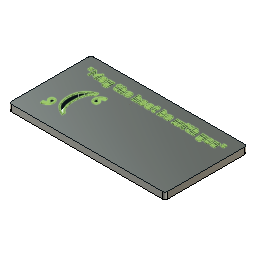
YodaHeatBot_dvirka (Autodesk Fusion 360 design; units mm, degrees)
Autodesk Fusion 360 part; units mm, degrees
(part 1 of 2)
sketch "Sketch1" plane through (0, 0, 0) normal (0, 0, 1) x (1, 0, 0)
  line L0 (-75, 65) -> (39, 65)
  line L1 (41, 63) -> (41, 5)
  line L2 (39, 3) -> (-75, 3)
  line L3 (-77, 5) -> (-77, 63)
  arc A0 (-75, 65) -> (-77, 63) centre (-75, 63) ccw
  arc A1 (41, 63) -> (39, 65) centre (39, 63) ccw
  arc A2 (39, 3) -> (41, 5) centre (39, 5) ccw
  arc A3 (-77, 5) -> (-75, 3) centre (-75, 5) ccw
  point P0 (-77, 65)
  point P1 (41, 65)
  point P2 (-77, 3)
  dimension "d1" = 118
  dimension "d2" = 62
  dimension "d3" = 2
  dimension "d4" = 2
  constraint horizontal L0
  constraint vertical L1
  constraint horizontal L2
  constraint vertical L3
  constraint coincident P0 L0
  constraint coincident P0 L3
  constraint tangent L0 A0
  constraint tangent L3 A0
  constraint coincident P1 L0
  constraint coincident P1 L1
  constraint tangent L0 A1
  constraint tangent L1 A1
  constraint equal A0 A1
  constraint tangent L1 A2
  constraint tangent L2 A2
  constraint equal A0 A2
  constraint coincident P2 L3
  constraint coincident P2 L2
  constraint tangent L3 A3
  constraint tangent L2 A3
  measures "d1" distance of P0 P1
  measures "d2" distance of P0 P2
  measures "d3" radius of A0
  measures "d4" radius of A3
extrude "Extrude1" add sketch "Sketch1" along normal blind 5
sketch "Sketch4" plane through (0, 0, 5) normal (0, 0, 1) x (-1, 0, 0)
  arc A0 (75, -65) -> (77, -63) centre (75, -63) ccw
  line L0 (77, -63) -> (77, -5)
  arc A1 (77, -5) -> (75, -3) centre (75, -5) ccw
  line L1 (75, -3) -> (-39, -3)
  arc A2 (-39, -3) -> (-41, -5) centre (-39, -5) ccw
  line L2 (-41, -5) -> (-41, -63)
  arc A3 (-41, -63) -> (-39, -65) centre (-39, -63) ccw
  line L3 (-39, -65) -> (75, -65)
  line L4 (49.3311, -42.4633) -> (49.3311, -41.8971)
  line L5 (49.3311, -41.8971) -> (49.3311, -41.4334)
  line L6 (49.3311, -41.4334) -> (49.3311, -41.1064)
  line L7 (49.3311, -41.1064) -> (49.3311, -40.8822)
  line L8 (49.3311, -40.8822) -> (49.3311, -40.7324)
  line L9 (49.3311, -40.7324) -> (49.3311, -40.6411)
  line L10 (49.3311, -40.6411) -> (49.3311, -40.6007)
  line L11 (49.3311, -40.6007) -> (49.7704, -40.287)
  line L12 (49.7704, -40.287) -> (50.1824, -39.9549)
  line L13 (50.1824, -39.9549) -> (50.5672, -39.6035)
  line L14 (50.5672, -39.6035) -> (50.9248, -39.2336)
  line L15 (50.9248, -39.2336) -> (51.256, -38.8444)
  line L16 (51.256, -38.8444) -> (51.5592, -38.4367)
  line L17 (51.5592, -38.4367) -> (51.8267, -38.0212)
  line L18 (51.8267, -38.0212) -> (51.8324, -38.0124)
  line L19 (51.8324, -38.0124) -> (52.0854, -37.574)
  line L20 (52.0854, -37.574) -> (52.3183, -37.1206)
  line L21 (52.3183, -37.1206) -> (52.5309, -36.6541)
  line L22 (52.5309, -36.6541) -> (52.7233, -36.1726)
  line L23 (52.7233, -36.1726) -> (52.8964, -35.678)
  line L24 (52.8964, -35.678) -> (53.0369, -35.2137)
  line L25 (53.0369, -35.2137) -> (53.0501, -35.1701)
  line L26 (53.0501, -35.1701) -> (53.1863, -34.6518)
  line L27 (53.1863, -34.6518) -> (53.2378, -34.4225)
  line L28 (53.2378, -34.4225) -> (53.3049, -34.1237)
  line L29 (53.3049, -34.1237) -> (53.4051, -33.5843)
  line L30 (53.4051, -33.5843) -> (53.4885, -33.0343)
  line L31 (53.4885, -33.0343) -> (53.5536, -32.4738)
  line L32 (53.5536, -32.4738) -> (53.6124, -31.9123)
  line L33 (53.6124, -31.9123) -> (53.6599, -31.3465)
  line L34 (53.6599, -31.3465) -> (53.6944, -30.8238)
  line L35 (53.6944, -30.8238) -> (53.6976, -30.7754)
  line L36 (53.6976, -30.7754) -> (53.724, -30.2008)
  line L37 (53.724, -30.2008) -> (53.7398, -29.6201)
  line L38 (53.7398, -29.6201) -> (53.7451, -29.0358)
  line L39 (53.7451, -29.0358) -> (53.7398, -28.4507)
  line L40 (53.7398, -28.4507) -> (53.724, -27.8708)
  line L41 (53.724, -27.8708) -> (53.6976, -27.2953)
  line L42 (53.6976, -27.2953) -> (53.693, -27.2251)
  line L43 (53.693, -27.2251) -> (53.6599, -26.7251)
  line L44 (53.6599, -26.7251) -> (53.6124, -26.1593)
  line L45 (53.6124, -26.1593) -> (53.5536, -25.5979)
  line L46 (53.5536, -25.5979) -> (53.4885, -25.0444)
  line L47 (53.4885, -25.0444) -> (53.4051, -24.5014)
  line L48 (53.4051, -24.5014) -> (53.3049, -23.969)
  line L49 (53.3049, -23.969) -> (53.2269, -23.6264)
  line L50 (53.2269, -23.6264) -> (53.1863, -23.448)
  line L51 (53.1863, -23.448) -> (53.0501, -22.9367)
  line L52 (53.0501, -22.9367) -> (53.0369, -22.8937)
  line L53 (53.0369, -22.8937) -> (52.8964, -22.4359)
  line L54 (52.8964, -22.4359) -> (52.7233, -21.9412)
  line L55 (52.7233, -21.9412) -> (52.5309, -21.4598)
  line L56 (52.5309, -21.4598) -> (52.3183, -20.9932)
  line L57 (52.3183, -20.9932) -> (52.0854, -20.5407)
  line L58 (52.0854, -20.5407) -> (51.8324, -20.1015)
  line L59 (51.8324, -20.1015) -> (51.7849, -20.0277)
  line L60 (51.7849, -20.0277) -> (51.5592, -19.6771)
  line L61 (51.5592, -19.6771) -> (51.256, -19.2633)
  line L62 (51.256, -19.2633) -> (50.9248, -18.8714)
  line L63 (50.9248, -18.8714) -> (50.5672, -18.4998)
  line L64 (50.5672, -18.4998) -> (50.1824, -18.1492)
  line L65 (50.1824, -18.1492) -> (49.7704, -17.8206)
  line L66 (49.7704, -17.8206) -> (49.3311, -17.5131)
  line L67 (49.3311, -17.5131) -> (49.3311, -16.4289)
  line L68 (49.3311, -16.4289) -> (49.3311, -15.6452)
  line L69 (49.3311, -15.6452) -> (50.1253, -15.9809)
  line L70 (50.1253, -15.9809) -> (50.88, -16.3367)
  line L71 (50.88, -16.3367) -> (51.0561, -16.4289)
  line L72 (51.0561, -16.4289) -> (51.5961, -16.7119)
  line L73 (51.5961, -16.7119) -> (52.2735, -17.1072)
  line L74 (52.2735, -17.1072) -> (52.9122, -17.5228)
  line L75 (52.9122, -17.5228) -> (53.0369, -17.6135)
  line L76 (53.0369, -17.6135) -> (53.5114, -17.9586)
  line L77 (53.5114, -17.9586) -> (54.0737, -18.4075)
  line L78 (54.0737, -18.4075) -> (54.6008, -18.8758)
  line L79 (54.6008, -18.8758) -> (55.0928, -19.3643)
  line L80 (55.0928, -19.3643) -> (55.5488, -19.873)
  line L81 (55.5488, -19.873) -> (55.9697, -20.4019)
  line L82 (55.9697, -20.4019) -> (56.3554, -20.951)
  line L83 (56.3554, -20.951) -> (56.7068, -21.5133)
  line L84 (56.7068, -21.5133) -> (57.0249, -22.0967)
  line L85 (57.0249, -22.0967) -> (57.3104, -22.7012)
  line L86 (57.3104, -22.7012) -> (57.5626, -23.3276)
  line L87 (57.5626, -23.3276) -> (57.6636, -23.6264)
  line L88 (57.6636, -23.6264) -> (57.7813, -23.9743)
  line L89 (57.7813, -23.9743) -> (57.9676, -24.6429)
  line L90 (57.9676, -24.6429) -> (58.1231, -25.3247)
  line L91 (58.1231, -25.3247) -> (58.2505, -26.0275)
  line L92 (58.2505, -26.0275) -> (58.3498, -26.7489)
  line L93 (58.3498, -26.7489) -> (58.3954, -27.2251)
  line L94 (58.3954, -27.2251) -> (58.4209, -27.4913)
  line L95 (58.4209, -27.4913) -> (58.4631, -28.2539)
  line L96 (58.4631, -28.2539) -> (58.4772, -29.0358)
  line L97 (58.4772, -29.0358) -> (58.4631, -29.8248)
  line L98 (58.4631, -29.8248) -> (58.4209, -30.5918)
  line L99 (58.4209, -30.5918) -> (58.3988, -30.8238)
  line L100 (58.3988, -30.8238) -> (58.3498, -31.3386)
  line L101 (58.3498, -31.3386) -> (58.2505, -32.0634)
  line L102 (58.2505, -32.0634) -> (58.1231, -32.7672)
  line L103 (58.1231, -32.7672) -> (57.9676, -33.4499)
  line L104 (57.9676, -33.4499) -> (57.7813, -34.1185)
  line L105 (57.7813, -34.1185) -> (57.6789, -34.4225)
  line L106 (57.6789, -34.4225) -> (57.5626, -34.7677)
  line L107 (57.5626, -34.7677) -> (57.3104, -35.3968)
  line L108 (57.3104, -35.3968) -> (57.0249, -36.0057)
  line L109 (57.0249, -36.0057) -> (56.7068, -36.5943)
  line L110 (56.7068, -36.5943) -> (56.3554, -37.1637)
  line L111 (56.3554, -37.1637) -> (55.9697, -37.7119)
  line L112 (55.9697, -37.7119) -> (55.7236, -38.0212)
  line L113 (55.7236, -38.0212) -> (55.5488, -38.2408)
  line L114 (55.5488, -38.2408) -> (55.0928, -38.7495)
  line L115 (55.0928, -38.7495) -> (54.6008, -39.238)
  line L116 (54.6008, -39.238) -> (54.0737, -39.7072)
  line L117 (54.0737, -39.7072) -> (53.5114, -40.1553)
  line L118 (53.5114, -40.1553) -> (53.0369, -40.501)
  line L119 (53.0369, -40.501) -> (52.9122, -40.5919)
  line L120 (52.9122, -40.5919) -> (52.2735, -41.0092)
  line L121 (52.2735, -41.0092) -> (51.5961, -41.4072)
  line L122 (51.5961, -41.4072) -> (50.88, -41.7868)
  line L123 (50.88, -41.7868) -> (50.1253, -42.1479)
  line L124 (50.1253, -42.1479) -> (49.3311, -42.4897)
  line L125 (49.3311, -42.4897) -> (49.3311, -42.4633)
  line L126 (64.1054, -21.6205) -> (64.0263, -21.8358)
  line L127 (64.0263, -21.8358) -> (63.92, -22.0273)
  line L128 (63.92, -22.0273) -> (63.8331, -22.1381)
  line L129 (63.8331, -22.1381) -> (63.7882, -22.1951)
  line L130 (63.7882, -22.1951) -> (63.6301, -22.3392)
  line L131 (63.6301, -22.3392) -> (63.4474, -22.464)
  line L132 (63.4474, -22.464) -> (63.2523, -22.5633)
  line L133 (63.2523, -22.5633) -> (63.0467, -22.6379)
  line L134 (63.0467, -22.6379) -> (62.8297, -22.688)
  line L135 (62.8297, -22.688) -> (62.6013, -22.7126)
  line L136 (62.6013, -22.7126) -> (62.3614, -22.7126)
  line L137 (62.3614, -22.7126) -> (62.0337, -22.6753)
  line L138 (62.0337, -22.6753) -> (62.0293, -22.6748)
  line L139 (62.0293, -22.6748) -> (61.7218, -22.5984)
  line L140 (61.7218, -22.5984) -> (61.4407, -22.4833)
  line L141 (61.4407, -22.4833) -> (61.185, -22.3296)
  line L142 (61.185, -22.3296) -> (60.9548, -22.1371)
  line L143 (60.9548, -22.1371) -> (60.7492, -21.9061)
  line L144 (60.7492, -21.9061) -> (60.5752, -21.6425)
  line L145 (60.5752, -21.6425) -> (60.4364, -21.3499)
  line L146 (60.4364, -21.3499) -> (60.3336, -21.031)
  line L147 (60.3336, -21.031) -> (60.266, -20.6848)
  line L148 (60.266, -20.6848) -> (60.2344, -20.3106)
  line L149 (60.2344, -20.3106) -> (60.2368, -20.0277)
  line L150 (60.2368, -20.0277) -> (60.2379, -19.909)
  line L151 (60.2379, -19.909) -> (60.259, -19.6534)
  line L152 (60.259, -19.6534) -> (60.2923, -19.4012)
  line L153 (60.2923, -19.4012) -> (60.3398, -19.1535)
  line L154 (60.3398, -19.1535) -> (60.4004, -18.9083)
  line L155 (60.4004, -18.9083) -> (60.4742, -18.6676)
  line L156 (60.4742, -18.6676) -> (60.5621, -18.4304)
  line L157 (60.5621, -18.4304) -> (60.6505, -18.2283)
  line L158 (60.6505, -18.2283) -> (60.664, -18.1976)
  line L159 (60.664, -18.1976) -> (60.78, -17.9726)
  line L160 (60.78, -17.9726) -> (60.91, -17.753)
  line L161 (60.91, -17.753) -> (61.0541, -17.5412)
  line L162 (61.0541, -17.5412) -> (61.2131, -17.3348)
  line L163 (61.2131, -17.3348) -> (61.3862, -17.1362)
  line L164 (61.3862, -17.1362) -> (61.5812, -16.9438)
  line L165 (61.5812, -16.9438) -> (61.7912, -16.7584)
  line L166 (61.7912, -16.7584) -> (62.0188, -16.5801)
  line L167 (62.0188, -16.5801) -> (62.0337, -16.5695)
  line L168 (62.0337, -16.5695) -> (62.2316, -16.4289)
  line L169 (62.2316, -16.4289) -> (62.2613, -16.4079)
  line L170 (62.2613, -16.4079) -> (62.5213, -16.2427)
  line L171 (62.5213, -16.2427) -> (62.7963, -16.0837)
  line L172 (62.7963, -16.0837) -> (63.095, -15.9405)
  line L173 (63.095, -15.9405) -> (63.4113, -15.8069)
  line L174 (63.4113, -15.8069) -> (63.7461, -15.6848)
  line L175 (63.7461, -15.6848) -> (64.0984, -15.5732)
  line L176 (64.0984, -15.5732) -> (64.4683, -15.4722)
  line L177 (64.4683, -15.4722) -> (64.8566, -15.3826)
  line L178 (64.8566, -15.3826) -> (64.802, -16.4289)
  line L179 (64.802, -16.4289) -> (64.7939, -16.5848)
  line L180 (64.7939, -16.5848) -> (64.7932, -16.5985)
  line L181 (64.7932, -16.5985) -> (64.7924, -16.6144)
  line L182 (64.7924, -16.6144) -> (64.7916, -16.6285)
  line L183 (64.7916, -16.6285) -> (64.7912, -16.6367)
  line L184 (64.7912, -16.6367) -> (64.7908, -16.6436)
  line L185 (64.7908, -16.6436) -> (64.7907, -16.646)
  line L186 (64.7907, -16.646) -> (64.615, -16.7013)
  line L187 (64.615, -16.7013) -> (64.4463, -16.7567)
  line L188 (64.4463, -16.7567) -> (64.2846, -16.8129)
  line L189 (64.2846, -16.8129) -> (64.13, -16.8691)
  line L190 (64.13, -16.8691) -> (63.9815, -16.9262)
  line L191 (63.9815, -16.9262) -> (63.8401, -16.9833)
  line L192 (63.8401, -16.9833) -> (63.8331, -16.9863)
  line L193 (63.8331, -16.9863) -> (63.7118, -17.0369)
  line L194 (63.7118, -17.0369) -> (63.5879, -17.0932)
  line L195 (63.5879, -17.0932) -> (63.4711, -17.1529)
  line L196 (63.4711, -17.1529) -> (63.3586, -17.2162)
  line L197 (63.3586, -17.2162) -> (63.2532, -17.2821)
  line L198 (63.2532, -17.2821) -> (63.1854, -17.3286)
  line L199 (63.1854, -17.3286) -> (63.1521, -17.3515)
  line L200 (63.1521, -17.3515) -> (63.0643, -17.4191)
  line L201 (63.0643, -17.4191) -> (62.9826, -17.4912)
  line L202 (62.9826, -17.4912) -> (62.9079, -17.5676)
  line L203 (62.9079, -17.5676) -> (62.8394, -17.6484)
  line L204 (62.8394, -17.6484) -> (62.7779, -17.7328)
  line L205 (62.7779, -17.7328) -> (62.7234, -17.8224)
  line L206 (62.7234, -17.8224) -> (62.6751, -17.9103)
  line L207 (62.6751, -17.9103) -> (62.6355, -18.0034)
  line L208 (62.6355, -18.0034) -> (62.603, -18.1018)
  line L209 (62.603, -18.1018) -> (62.5775, -18.2055)
  line L210 (62.5775, -18.2055) -> (62.574, -18.2283)
  line L211 (62.574, -18.2283) -> (62.5609, -18.3144)
  line L212 (62.5609, -18.3144) -> (62.5503, -18.4286)
  line L213 (62.5503, -18.4286) -> (62.5503, -18.5033)
  line L214 (62.5503, -18.5033) -> (62.5582, -18.5736)
  line L215 (62.5582, -18.5736) -> (62.5749, -18.6412)
  line L216 (62.5749, -18.6412) -> (62.5986, -18.7054)
  line L217 (62.5986, -18.7054) -> (62.6303, -18.7651)
  line L218 (62.6303, -18.7651) -> (62.6707, -18.8222)
  line L219 (62.6707, -18.8222) -> (62.712, -18.8705)
  line L220 (62.712, -18.8705) -> (62.7577, -18.9189)
  line L221 (62.7577, -18.9189) -> (62.8086, -18.9654)
  line L222 (62.8086, -18.9654) -> (62.864, -19.012)
  line L223 (62.864, -19.012) -> (62.8834, -19.0266)
  line L224 (62.8834, -19.0266) -> (62.9246, -19.0577)
  line L225 (62.9246, -19.0577) -> (62.9905, -19.1025)
  line L226 (62.9905, -19.1025) -> (63.0265, -19.128)
  line L227 (63.0265, -19.128) -> (63.0537, -19.1473)
  line L228 (63.0537, -19.1473) -> (63.072, -19.1604)
  line L229 (63.072, -19.1604) -> (63.1188, -19.1939)
  line L230 (63.1188, -19.1939) -> (63.1855, -19.2404)
  line L231 (63.1855, -19.2404) -> (63.2273, -19.2699)
  line L232 (63.2273, -19.2699) -> (63.2541, -19.2888)
  line L233 (63.2541, -19.2888) -> (63.3252, -19.338)
  line L234 (63.3252, -19.338) -> (63.3973, -19.388)
  line L235 (63.3973, -19.388) -> (63.4702, -19.4408)
  line L236 (63.4702, -19.4408) -> (63.5405, -19.497)
  line L237 (63.5405, -19.497) -> (63.609, -19.5576)
  line L238 (63.609, -19.5576) -> (63.6749, -19.6217)
  line L239 (63.6749, -19.6217) -> (63.739, -19.6894)
  line L240 (63.739, -19.6894) -> (63.8005, -19.7614)
  line L241 (63.8005, -19.7614) -> (63.8331, -19.8002)
  line L242 (63.8331, -19.8002) -> (63.8647, -19.8379)
  line L243 (63.8647, -19.8379) -> (63.9227, -19.9205)
  line L244 (63.9227, -19.9205) -> (63.9763, -20.0083)
  line L245 (63.9763, -20.0083) -> (63.9863, -20.0277)
  line L246 (63.9863, -20.0277) -> (64.0246, -20.1015)
  line L247 (64.0246, -20.1015) -> (64.0685, -20.2007)
  line L248 (64.0685, -20.2007) -> (64.1063, -20.3053)
  line L249 (64.1063, -20.3053) -> (64.1379, -20.4169)
  line L250 (64.1379, -20.4169) -> (64.1625, -20.539)
  line L251 (64.1625, -20.539) -> (64.1792, -20.6699)
  line L252 (64.1792, -20.6699) -> (64.1889, -20.8096)
  line L253 (64.1889, -20.8096) -> (64.1915, -20.9598)
  line L254 (64.1915, -20.9598) -> (64.1871, -21.1189)
  line L255 (64.1871, -21.1189) -> (64.159, -21.3816)
  line L256 (64.159, -21.3816) -> (64.1054, -21.6205)
  line L257 (46.9466, -38.7091) -> (46.8851, -38.9533)
  line L258 (46.8851, -38.9533) -> (46.8095, -39.195)
  line L259 (46.8095, -39.195) -> (46.7199, -39.4322)
  line L260 (46.7199, -39.4322) -> (46.6162, -39.6632)
  line L261 (46.6162, -39.6632) -> (46.4976, -39.889)
  line L262 (46.4976, -39.889) -> (46.3641, -40.1087)
  line L263 (46.3641, -40.1087) -> (46.2165, -40.3222)
  line L264 (46.2165, -40.3222) -> (46.0539, -40.5304)
  line L265 (46.0539, -40.5304) -> (45.8703, -40.7325)
  line L266 (45.8703, -40.7325) -> (45.8395, -40.7624)
  line L267 (45.8395, -40.7624) -> (45.6691, -40.9284)
  line L268 (45.6691, -40.9284) -> (45.4521, -41.1191)
  line L269 (45.4521, -41.1191) -> (45.2184, -41.3036)
  line L270 (45.2184, -41.3036) -> (44.968, -41.4819)
  line L271 (44.968, -41.4819) -> (44.7551, -41.6199)
  line L272 (44.7551, -41.6199) -> (44.7009, -41.655)
  line L273 (44.7009, -41.655) -> (44.4101, -41.814)
  line L274 (44.4101, -41.814) -> (44.1017, -41.9634)
  line L275 (44.1017, -41.9634) -> (43.774, -42.1031)
  line L276 (43.774, -42.1031) -> (43.4278, -42.2331)
  line L277 (43.4278, -42.2331) -> (43.0632, -42.3526)
  line L278 (43.0632, -42.3526) -> (42.6801, -42.4633)
  line L279 (42.6801, -42.4633) -> (42.6801, -41.6199)
  line L280 (42.6801, -41.6199) -> (42.6801, -41.4417)
  line L281 (42.6801, -41.4417) -> (42.6801, -41.3678)
  line L282 (42.6801, -41.3678) -> (42.6801, -41.3073)
  line L283 (42.6801, -41.3073) -> (42.6801, -41.2544)
  line L284 (42.6801, -41.2544) -> (42.6801, -41.2446)
  line L285 (42.6801, -41.2446) -> (42.6801, -41.2315)
  line L286 (42.6801, -41.2315) -> (42.6801, -41.2143)
  line L287 (42.6801, -41.2143) -> (42.6801, -41.2051)
  line L288 (42.6801, -41.2051) -> (42.6801, -41.2018)
  line L289 (42.6801, -41.2018) -> (42.6801, -41.1981)
  line L290 (42.6801, -41.1981) -> (42.8523, -41.134)
  line L291 (42.8523, -41.134) -> (43.0175, -41.069)
  line L292 (43.0175, -41.069) -> (43.1765, -41.0049)
  line L293 (43.1765, -41.0049) -> (43.3285, -40.9407)
  line L294 (43.3285, -40.9407) -> (43.4735, -40.8757)
  line L295 (43.4735, -40.8757) -> (43.6114, -40.8116)
  line L296 (43.6114, -40.8116) -> (43.7371, -40.7518)
  line L297 (43.7371, -40.7518) -> (43.8574, -40.6886)
  line L298 (43.8574, -40.6886) -> (43.9717, -40.6227)
  line L299 (43.9717, -40.6227) -> (44.0402, -40.5792)
  line L300 (44.0402, -40.5792) -> (44.0797, -40.5541)
  line L301 (44.0797, -40.5541) -> (44.1825, -40.4821)
  line L302 (44.1825, -40.4821) -> (44.2792, -40.4074)
  line L303 (44.2792, -40.4074) -> (44.3635, -40.3354)
  line L304 (44.3635, -40.3354) -> (44.4408, -40.2589)
  line L305 (44.4408, -40.2589) -> (44.512, -40.179)
  line L306 (44.512, -40.179) -> (44.5761, -40.0946)
  line L307 (44.5761, -40.0946) -> (44.6332, -40.0068)
  line L308 (44.6332, -40.0068) -> (44.6833, -39.9154)
  line L309 (44.6833, -39.9154) -> (44.7264, -39.8249)
  line L310 (44.7264, -39.8249) -> (44.728, -39.8205)
  line L311 (44.728, -39.8205) -> (44.7615, -39.73)
  line L312 (44.7615, -39.73) -> (44.7887, -39.6299)
  line L313 (44.7887, -39.6299) -> (44.8081, -39.5253)
  line L314 (44.8081, -39.5253) -> (44.8204, -39.4155)
  line L315 (44.8204, -39.4155) -> (44.8239, -39.3004)
  line L316 (44.8239, -39.3004) -> (44.8204, -39.2266)
  line L317 (44.8204, -39.2266) -> (44.8081, -39.1563)
  line L318 (44.8081, -39.1563) -> (44.7887, -39.0895)
  line L319 (44.7887, -39.0895) -> (44.7615, -39.0271)
  line L320 (44.7615, -39.0271) -> (44.7264, -38.9683)
  line L321 (44.7264, -38.9683) -> (44.6889, -38.9208)
  line L322 (44.6889, -38.9208) -> (44.6833, -38.9138)
  line L323 (44.6833, -38.9138) -> (44.6403, -38.8672)
  line L324 (44.6403, -38.8672) -> (44.5919, -38.8224)
  line L325 (44.5919, -38.8224) -> (44.5384, -38.7776)
  line L326 (44.5384, -38.7776) -> (44.4804, -38.7346)
  line L327 (44.4804, -38.7346) -> (44.454, -38.7166)
  line L328 (44.454, -38.7166) -> (44.4395, -38.7067)
  line L329 (44.4395, -38.7067) -> (44.4171, -38.6915)
  line L330 (44.4171, -38.6915) -> (44.3579, -38.6554)
  line L331 (44.3579, -38.6554) -> (44.3495, -38.6502)
  line L332 (44.3495, -38.6502) -> (44.3199, -38.6315)
  line L333 (44.3199, -38.6315) -> (44.2844, -38.6089)
  line L334 (44.2844, -38.6089) -> (44.2168, -38.5659)
  line L335 (44.2168, -38.5659) -> (44.1474, -38.5228)
  line L336 (44.1474, -38.5228) -> (44.0762, -38.478)
  line L337 (44.0762, -38.478) -> (44.0402, -38.4559)
  line L338 (44.0402, -38.4559) -> (44.0033, -38.4332)
  line L339 (44.0033, -38.4332) -> (43.9277, -38.3867)
  line L340 (43.9277, -38.3867) -> (43.8522, -38.3375)
  line L341 (43.8522, -38.3375) -> (43.7792, -38.2847)
  line L342 (43.7792, -38.2847) -> (43.7081, -38.2285)
  line L343 (43.7081, -38.2285) -> (43.6387, -38.1679)
  line L344 (43.6387, -38.1679) -> (43.571, -38.1038)
  line L345 (43.571, -38.1038) -> (43.506, -38.0352)
  line L346 (43.506, -38.0352) -> (43.493, -38.0212)
  line L347 (43.493, -38.0212) -> (43.4384, -37.9623)
  line L348 (43.4384, -37.9623) -> (43.3751, -37.8832)
  line L349 (43.3751, -37.8832) -> (43.3171, -37.798)
  line L350 (43.3171, -37.798) -> (43.2635, -37.7075)
  line L351 (43.2635, -37.7075) -> (43.2152, -37.6109)
  line L352 (43.2152, -37.6109) -> (43.1721, -37.5081)
  line L353 (43.1721, -37.5081) -> (43.1344, -37.3974)
  line L354 (43.1344, -37.3974) -> (43.1036, -37.2779)
  line L355 (43.1036, -37.2779) -> (43.0799, -37.1478)
  line L356 (43.0799, -37.1478) -> (43.0632, -37.0082)
  line L357 (43.0632, -37.0082) -> (43.0527, -36.8588)
  line L358 (43.0527, -36.8588) -> (43.0491, -36.6998)
  line L359 (43.0491, -36.6998) -> (43.0632, -36.4353)
  line L360 (43.0632, -36.4353) -> (43.0989, -36.2218)
  line L361 (43.0989, -36.2218) -> (43.1036, -36.1937)
  line L362 (43.1036, -36.1937) -> (43.1721, -35.9749)
  line L363 (43.1721, -35.9749) -> (43.2679, -35.7781)
  line L364 (43.2679, -35.7781) -> (43.3909, -35.6042)
  line L365 (43.3909, -35.6042) -> (43.5412, -35.4522)
  line L366 (43.5412, -35.4522) -> (43.7177, -35.3177)
  line L367 (43.7177, -35.3177) -> (43.9066, -35.2079)
  line L368 (43.9066, -35.2079) -> (44.0402, -35.1514)
  line L369 (44.0402, -35.1514) -> (44.1078, -35.1227)
  line L370 (44.1078, -35.1227) -> (44.3222, -35.0621)
  line L371 (44.3222, -35.0621) -> (44.5489, -35.0252)
  line L372 (44.5489, -35.0252) -> (44.7887, -35.0129)
  line L373 (44.7887, -35.0129) -> (45.1226, -35.0331)
  line L374 (45.1226, -35.0331) -> (45.4328, -35.0928)
  line L375 (45.4328, -35.0928) -> (45.7201, -35.193)
  line L376 (45.7201, -35.193) -> (45.8395, -35.2563)
  line L377 (45.8395, -35.2563) -> (45.9836, -35.3327)
  line L378 (45.9836, -35.3327) -> (46.2235, -35.5128)
  line L379 (46.2235, -35.5128) -> (46.4405, -35.7333)
  line L380 (46.4405, -35.7333) -> (46.6285, -35.9881)
  line L381 (46.6285, -35.9881) -> (46.7823, -36.2719)
  line L382 (46.7823, -36.2719) -> (46.9018, -36.5856)
  line L383 (46.9018, -36.5856) -> (46.987, -36.9282)
  line L384 (46.987, -36.9282) -> (47.0388, -37.2998)
  line L385 (47.0388, -37.2998) -> (47.0555, -37.7014)
  line L386 (47.0555, -37.7014) -> (47.0485, -37.9579)
  line L387 (47.0485, -37.9579) -> (47.0434, -38.0212)
  line L388 (47.0434, -38.0212) -> (47.0283, -38.2109)
  line L389 (47.0283, -38.2109) -> (46.994, -38.4613)
  line L390 (46.994, -38.4613) -> (46.9466, -38.7091)
  line L391 (68.8125, -55.0356) -> (68.8125, -56.7856)
  line L392 (68.8125, -56.7856) -> (68.2315, -56.7856)
  line L393 (68.2315, -56.7856) -> (68.2315, -55.0356)
  line L394 (68.2315, -55.0356) -> (68.8125, -55.0356)
  line L395 (67.6505, -55.0356) -> (67.6505, -56.7856)
  line L396 (67.6505, -56.7856) -> (67.0625, -56.7856)
  line L397 (67.0625, -56.7856) -> (67.0625, -55.0356)
  line L398 (67.0625, -55.0356) -> (67.6505, -55.0356)
  line L399 (65.3195, -51.5356) -> (65.3195, -56.7856)
  line L400 (65.3195, -56.7856) -> (65.0465, -56.7856)
  line L401 (65.0465, -56.7856) -> (62.5545, -54.3006)
  line L402 (62.5545, -54.3006) -> (60.0695, -56.7856)
  line L403 (60.0695, -56.7856) -> (59.4815, -56.7856)
  line L404 (59.4815, -56.7856) -> (59.4815, -51.5356)
  line L405 (59.4815, -51.5356) -> (60.6505, -51.5356)
  line L406 (60.6505, -51.5356) -> (60.6505, -54.7416)
  line L407 (60.6505, -54.7416) -> (62.6945, -52.6976)
  line L408 (62.6945, -52.6976) -> (64.7315, -54.7416)
  line L409 (64.7315, -54.7416) -> (64.7315, -51.5356)
  line L410 (64.7315, -51.5356) -> (65.3195, -51.5356)
  line L411 (55.9815, -53.8666) -> (55.9815, -54.4546)
  spline S0 degree 3 poles (55.9815, -54.4546) (55.9889, -54.5312) (56.0039, -54.6852) (56.1055, -54.8019) (56.1565, -54.8606) knots 0 0 0 0 0.02248 0.045204 0.045204 0.045204 0.045204
  spline S1 degree 3 poles (56.1565, -54.8606) (56.2158, -54.9117) (56.3348, -55.0141) (56.4911, -55.0284) (56.5695, -55.0356) knots 0 0 0 0 0.022867 0.045862 0.045862 0.045862 0.045862
  line L412 (56.5695, -55.0356) -> (57.1505, -55.0356)
  spline S2 degree 3 poles (57.1505, -55.0356) (57.3046, -55.0073) (57.6273, -54.9481) (57.6957, -54.624) (57.7315, -54.4546) knots 0 0 0 0 0.042955 0.089979 0.089979 0.089979 0.089979
  line L413 (57.7315, -54.4546) -> (58.3195, -54.4546)
  spline S3 degree 3 poles (58.3195, -54.4546) (58.2447, -54.7933) (58.1018, -55.4397) (57.4573, -55.5596) (57.1505, -55.6166) knots 0 0 0 0 0.094379 0.180125 0.180125 0.180125 0.180125
  line L414 (57.1505, -55.6166) -> (55.9815, -55.6166)
  spline S4 degree 3 poles (55.9815, -55.6166) (55.8281, -55.6021) (55.5196, -55.5727) (55.2819, -55.3737) (55.1625, -55.2736) knots 0 0 0 0 0.045098 0.090676 0.090676 0.090676 0.090676
  spline S5 degree 3 poles (55.1625, -55.2736) (55.0625, -55.1542) (54.8634, -54.9166) (54.8341, -54.6081) (54.8195, -54.4546) knots 0 0 0 0 0.045579 0.090676 0.090676 0.090676 0.090676
  line L415 (54.8195, -54.4546) -> (54.8195, -51.5356)
  line L416 (54.8195, -51.5356) -> (55.9815, -51.5356)
  line L417 (55.9815, -51.5356) -> (55.9815, -52.1166)
  spline S6 degree 3 poles (55.9815, -52.1166) (56.0193, -51.9473) (56.0916, -51.6233) (56.4151, -51.564) (56.5695, -51.5356) knots 0 0 0 0 0.047223 0.090343 0.090343 0.090343 0.090343
  line L418 (56.5695, -51.5356) -> (57.1505, -51.5356)
  spline S7 degree 3 poles (57.1505, -51.5356) (57.3044, -51.5504) (57.6147, -51.5801) (57.8552, -51.7786) (57.9765, -51.8786) knots 0 0 0 0 0.04527 0.091283 0.091283 0.091283 0.091283
  spline S8 degree 3 poles (57.9765, -51.8786) (58.0765, -51.9987) (58.2764, -52.2386) (58.3051, -52.5494) (58.3195, -52.7046) knots 0 0 0 0 0.045723 0.091337 0.091337 0.091337 0.091337
  spline S9 degree 3 poles (58.3195, -52.7046) (58.3049, -52.8581) (58.2756, -53.1666) (58.0765, -53.4042) (57.9765, -53.5236) knots 0 0 0 0 0.045098 0.090676 0.090676 0.090676 0.090676
  spline S10 degree 3 poles (57.9765, -53.5236) (57.8552, -53.6237) (57.6147, -53.8222) (57.3044, -53.8519) (57.1505, -53.8666) knots 0 0 0 0 0.046013 0.091283 0.091283 0.091283 0.091283
  line L419 (57.1505, -53.8666) -> (55.9815, -53.8666)
  line L420 (55.9815, -53.2856) -> (56.5695, -53.2856)
  spline S11 degree 3 poles (56.5695, -53.2856) (56.6465, -53.278) (56.8023, -53.2627) (56.922, -53.1617) (56.9825, -53.1106) knots 0 0 0 0 0.022652 0.045806 0.045806 0.045806 0.045806
  spline S12 degree 3 poles (56.9825, -53.1106) (57.0315, -53.0517) (57.1295, -52.9338) (57.1435, -52.7811) (57.1505, -52.7046) knots 0 0 0 0 0.022425 0.044871 0.044871 0.044871 0.044871
  spline S13 degree 3 poles (57.1505, -52.7046) (57.1433, -52.6278) (57.129, -52.4732) (57.0315, -52.3524) (56.9825, -52.2916) knots 0 0 0 0 0.022618 0.045479 0.045479 0.045479 0.045479
  spline S14 degree 3 poles (56.9825, -52.2916) (56.922, -52.2406) (56.8023, -52.1396) (56.6465, -52.1243) (56.5695, -52.1166) knots 0 0 0 0 0.023154 0.045806 0.045806 0.045806 0.045806
  spline S15 degree 3 poles (56.5695, -52.1166) (56.4911, -52.1239) (56.3348, -52.1382) (56.2158, -52.2406) (56.1565, -52.2916) knots 0 0 0 0 0.022995 0.045862 0.045862 0.045862 0.045862
  spline S16 degree 3 poles (56.1565, -52.2916) (56.1055, -52.3522) (56.0045, -52.4719) (55.9891, -52.6276) (55.9815, -52.7046) knots 0 0 0 0 0.023154 0.045806 0.045806 0.045806 0.045806
  line L421 (55.9815, -52.7046) -> (55.9815, -53.2856)
  spline S17 degree 3 poles (53.0625, -50.9546) (53.031, -50.7832) (52.9702, -50.4517) (52.6406, -50.3943) (52.4815, -50.3666) knots 0 0 0 0 0.04713 0.091133 0.091133 0.091133 0.091133
  line L422 (52.4815, -50.3666) -> (51.9005, -50.3666)
  spline S18 degree 3 poles (51.9005, -50.3666) (51.8221, -50.3739) (51.6658, -50.3882) (51.5468, -50.4906) (51.4875, -50.5416) knots 0 0 0 0 0.022995 0.045862 0.045862 0.045862 0.045862
  spline S19 degree 3 poles (51.4875, -50.5416) (51.4365, -50.601) (51.3341, -50.7199) (51.3197, -50.8763) (51.3125, -50.9546) knots 0 0 0 0 0.022867 0.045862 0.045862 0.045862 0.045862
  line L423 (51.3125, -50.9546) -> (51.3125, -52.1166)
  spline S20 degree 3 poles (51.3125, -52.1166) (51.3503, -51.9473) (51.4226, -51.6233) (51.7461, -51.564) (51.9005, -51.5356) knots 0 0 0 0 0.047223 0.090343 0.090343 0.090343 0.090343
  line L424 (51.9005, -51.5356) -> (52.4815, -51.5356)
  spline S21 degree 3 poles (52.4815, -51.5356) (52.6354, -51.5504) (52.9457, -51.5801) (53.1862, -51.7786) (53.3075, -51.8786) knots 0 0 0 0 0.04527 0.091283 0.091283 0.091283 0.091283
  spline S22 degree 3 poles (53.3075, -51.8786) (53.4075, -51.9987) (53.6074, -52.2386) (53.6361, -52.5494) (53.6505, -52.7046) knots 0 0 0 0 0.045723 0.091336 0.091336 0.091336 0.091336
  line L425 (53.6505, -52.7046) -> (53.6505, -55.6166)
  line L426 (53.6505, -55.6166) -> (52.4815, -55.6166)
  line L427 (52.4815, -55.6166) -> (52.4815, -52.7046)
  spline S23 degree 3 poles (52.4815, -52.7046) (52.4743, -52.6278) (52.46, -52.4732) (52.3625, -52.3524) (52.3135, -52.2916) knots 0 0 0 0 0.022618 0.045479 0.045479 0.045479 0.045479
  spline S24 degree 3 poles (52.3135, -52.2916) (52.253, -52.2406) (52.1333, -52.1396) (51.9775, -52.1243) (51.9005, -52.1166) knots 0 0 0 0 0.023154 0.045806 0.045806 0.045806 0.045806
  spline S25 degree 3 poles (51.9005, -52.1166) (51.8221, -52.1239) (51.6658, -52.1382) (51.5468, -52.2406) (51.4875, -52.2916) knots 0 0 0 0 0.022995 0.045862 0.045862 0.045862 0.045862
  spline S26 degree 3 poles (51.4875, -52.2916) (51.4365, -52.3522) (51.3355, -52.4719) (51.3201, -52.6276) (51.3125, -52.7046) knots 0 0 0 0 0.023154 0.045806 0.045806 0.045806 0.045806
  line L428 (51.3125, -52.7046) -> (51.3125, -55.6166)
  line L429 (51.3125, -55.6166) -> (50.1505, -55.6166)
  line L430 (50.1505, -55.6166) -> (50.1505, -50.9546)
  spline S27 degree 3 poles (50.1505, -50.9546) (50.1651, -50.8012) (50.1944, -50.4927) (50.3935, -50.2551) (50.4935, -50.1356) knots 0 0 0 0 0.045098 0.090676 0.090676 0.090676 0.090676
  spline S28 degree 3 poles (50.4935, -50.1356) (50.6127, -50.0336) (50.8492, -49.8311) (51.1589, -49.8007) (51.3125, -49.7856) knots 0 0 0 0 0.045877 0.091008 0.091008 0.091008 0.091008
  line L431 (51.3125, -49.7856) -> (52.4815, -49.7856)
  spline S29 degree 3 poles (52.4815, -49.7856) (52.7883, -49.8434) (53.4344, -49.9651) (53.5761, -50.6139) (53.6505, -50.9546) knots 0 0 0 0 0.085805 0.180669 0.180669 0.180669 0.180669
  line L432 (53.6505, -50.9546) -> (53.0625, -50.9546)
  line L433 (46.6435, -56.7856) -> (45.4815, -56.7856)
  line L434 (45.4815, -56.7856) -> (45.4815, -55.6166)
  line L435 (45.4815, -55.6166) -> (44.8935, -55.6166)
  line L436 (44.8935, -55.6166) -> (44.8935, -55.0356)
  line L437 (44.8935, -55.0356) -> (45.4815, -55.0356)
  line L438 (45.4815, -55.0356) -> (45.4815, -52.7046)
  spline S30 degree 3 poles (45.4815, -52.7046) (45.4752, -52.6159) (45.4632, -52.4463) (45.3476, -52.3226) (45.2925, -52.2636) knots 0 0 0 0 0.025811 0.049296 0.049296 0.049296 0.049296
  spline S31 degree 3 poles (45.2925, -52.2636) (45.2348, -52.221) (45.1316, -52.1446) (45.0052, -52.1252) (44.9495, -52.1166) knots 0 0 0 0 0.02113 0.037814 0.037814 0.037814 0.037814
  line L439 (44.9495, -52.1166) -> (44.8935, -52.1166)
  line L440 (44.8935, -52.1166) -> (44.8935, -51.5356)
  line L441 (44.8935, -51.5356) -> (45.4815, -51.5356)
  spline S32 degree 3 poles (45.4815, -51.5356) (45.6349, -51.5502) (45.9434, -51.5796) (46.181, -51.7786) (46.3005, -51.8786) knots 0 0 0 0 0.045098 0.090677 0.090677 0.090677 0.090677
  spline S33 degree 3 poles (46.3005, -51.8786) (46.4005, -51.9987) (46.6004, -52.2386) (46.6291, -52.5494) (46.6435, -52.7046) knots 0 0 0 0 0.045723 0.091337 0.091337 0.091337 0.091337
  line L442 (46.6435, -52.7046) -> (46.6435, -55.0356)
  line L443 (46.6435, -55.0356) -> (47.2315, -55.0356)
  line L444 (47.2315, -55.0356) -> (47.2315, -55.6166)
  line L445 (47.2315, -55.6166) -> (46.6435, -55.6166)
  line L446 (46.6435, -55.6166) -> (46.6435, -56.7856)
  line L447 (43.7315, -51.5356) -> (43.7315, -56.7856)
  line L448 (43.7315, -56.7856) -> (42.5625, -56.7856)
  line L449 (42.5625, -56.7856) -> (42.5625, -55.0356)
  spline S34 degree 3 poles (42.5625, -55.0356) (42.5491, -55.1242) (42.5248, -55.2849) (42.4252, -55.4124) (42.3805, -55.4696) knots 0 0 0 0 0.026315 0.047768 0.047768 0.047768 0.047768
  spline S35 degree 3 poles (42.3805, -55.4696) (42.3251, -55.5125) (42.2079, -55.603) (42.0596, -55.612) (41.9815, -55.6166) knots 0 0 0 0 0.020535 0.043408 0.043408 0.043408 0.043408
  line L450 (41.9815, -55.6166) -> (41.3935, -55.6166)
  spline S36 degree 3 poles (41.3935, -55.6166) (41.2401, -55.6021) (40.9316, -55.5727) (40.6939, -55.3737) (40.5745, -55.2736) knots 0 0 0 0 0.045098 0.090676 0.090676 0.090676 0.090676
  spline S37 degree 3 poles (40.5745, -55.2736) (40.4744, -55.1542) (40.2754, -54.9166) (40.2461, -54.6081) (40.2315, -54.4546) knots 0 0 0 0 0.045579 0.090676 0.090676 0.090676 0.090676
  line L451 (40.2315, -54.4546) -> (40.2315, -51.5356)
  line L452 (40.2315, -51.5356) -> (41.3935, -51.5356)
  line L453 (41.3935, -51.5356) -> (41.3935, -54.4546)
  spline S38 degree 3 poles (41.3935, -54.4546) (41.4009, -54.5312) (41.4159, -54.6852) (41.5174, -54.8019) (41.5685, -54.8606) knots 0 0 0 0 0.02248 0.045204 0.045204 0.045204 0.045204
  spline S39 degree 3 poles (41.5685, -54.8606) (41.6278, -54.9117) (41.7468, -55.0141) (41.9031, -55.0284) (41.9815, -55.0356) knots 0 0 0 0 0.022867 0.045862 0.045862 0.045862 0.045862
  spline S40 degree 3 poles (41.9815, -55.0356) (42.0585, -55.028) (42.2143, -55.0127) (42.334, -54.9117) (42.3945, -54.8606) knots 0 0 0 0 0.022652 0.045806 0.045806 0.045806 0.045806
  spline S41 degree 3 poles (42.3945, -54.8606) (42.4435, -54.8017) (42.5415, -54.6838) (42.5555, -54.5311) (42.5625, -54.4546) knots 0 0 0 0 0.022425 0.044871 0.044871 0.044871 0.044871
  line L454 (42.5625, -54.4546) -> (42.5625, -51.5356)
  line L455 (42.5625, -51.5356) -> (43.7315, -51.5356)
  line L456 (35.5625, -53.2856) -> (37.8935, -53.2856)
  line L457 (37.8935, -53.2856) -> (37.8935, -52.7046)
  spline S42 degree 3 poles (37.8935, -52.7046) (37.8863, -52.6278) (37.872, -52.4732) (37.7745, -52.3524) (37.7255, -52.2916) knots 0 0 0 0 0.022618 0.045479 0.045479 0.045479 0.045479
  spline S43 degree 3 poles (37.7255, -52.2916) (37.665, -52.2406) (37.5453, -52.1396) (37.3895, -52.1243) (37.3125, -52.1166) knots 0 0 0 0 0.023154 0.045806 0.045806 0.045806 0.045806
  line L458 (37.3125, -52.1166) -> (36.7245, -52.1166)
  spline S44 degree 3 poles (36.7245, -52.1166) (36.555, -52.1416) (36.2145, -52.1918) (36.1672, -52.5331) (36.1435, -52.7046) knots 0 0 0 0 0.045988 0.092418 0.092418 0.092418 0.092418
  line L459 (36.1435, -52.7046) -> (35.5625, -52.7046)
  spline S45 degree 3 poles (35.5625, -52.7046) (35.6349, -52.3639) (35.7727, -51.715) (36.418, -51.5934) (36.7245, -51.5356) knots 0 0 0 0 0.094665 0.180305 0.180305 0.180305 0.180305
  line L460 (36.7245, -51.5356) -> (37.8935, -51.5356)
  spline S46 degree 3 poles (37.8935, -51.5356) (38.0474, -51.5504) (38.3577, -51.5801) (38.5982, -51.7786) (38.7195, -51.8786) knots 0 0 0 0 0.04527 0.091283 0.091283 0.091283 0.091283
  spline S47 degree 3 poles (38.7195, -51.8786) (38.8195, -51.9987) (39.0194, -52.2386) (39.0481, -52.5494) (39.0625, -52.7046) knots 0 0 0 0 0.045723 0.091337 0.091337 0.091337 0.091337
  line L461 (39.0625, -52.7046) -> (39.0625, -54.4546)
  spline S48 degree 3 poles (39.0625, -54.4546) (39.0479, -54.6081) (39.0186, -54.9166) (38.8195, -55.1542) (38.7195, -55.2736) knots 0 0 0 0 0.045098 0.090676 0.090676 0.090676 0.090676
  spline S49 degree 3 poles (38.7195, -55.2736) (38.5982, -55.3737) (38.3577, -55.5722) (38.0474, -55.6019) (37.8935, -55.6166) knots 0 0 0 0 0.046013 0.091283 0.091283 0.091283 0.091283
  line L462 (37.8935, -55.6166) -> (36.7245, -55.6166)
  spline S50 degree 3 poles (36.7245, -55.6166) (36.5711, -55.6021) (36.2626, -55.5727) (36.0249, -55.3737) (35.9055, -55.2736) knots 0 0 0 0 0.045098 0.090676 0.090676 0.090676 0.090676
  spline S51 degree 3 poles (35.9055, -55.2736) (35.8055, -55.1542) (35.6064, -54.9166) (35.5771, -54.6081) (35.5625, -54.4546) knots 0 0 0 0 0.045579 0.090676 0.090676 0.090676 0.090676
  line L463 (35.5625, -54.4546) -> (35.5625, -53.2856)
  line L464 (37.8935, -53.8666) -> (36.7245, -53.8666)
  line L465 (36.7245, -53.8666) -> (36.7245, -54.4546)
  spline S52 degree 3 poles (36.7245, -54.4546) (36.7319, -54.5312) (36.7469, -54.6852) (36.8485, -54.8019) (36.8995, -54.8606) knots 0 0 0 0 0.02248 0.045204 0.045204 0.045204 0.045204
  spline S53 degree 3 poles (36.8995, -54.8606) (36.9588, -54.9117) (37.0778, -55.0141) (37.2341, -55.0284) (37.3125, -55.0356) knots 0 0 0 0 0.022867 0.045862 0.045862 0.045862 0.045862
  spline S54 degree 3 poles (37.3125, -55.0356) (37.3895, -55.028) (37.5453, -55.0127) (37.665, -54.9117) (37.7255, -54.8606) knots 0 0 0 0 0.022652 0.045806 0.045806 0.045806 0.045806
  spline S55 degree 3 poles (37.7255, -54.8606) (37.7745, -54.8017) (37.8725, -54.6838) (37.8865, -54.5311) (37.8935, -54.4546) knots 0 0 0 0 0.022425 0.044871 0.044871 0.044871 0.044871
  line L466 (37.8935, -54.4546) -> (37.8935, -53.8666)
  line L467 (32.6435, -51.5356) -> (32.6435, -56.7856)
  line L468 (32.6435, -56.7856) -> (31.4745, -56.7856)
  line L469 (31.4745, -56.7856) -> (31.4745, -55.0356)
  spline S56 degree 3 poles (31.4745, -55.0356) (31.4611, -55.1242) (31.4368, -55.2849) (31.3372, -55.4124) (31.2925, -55.4696) knots 0 0 0 0 0.026315 0.047768 0.047768 0.047768 0.047768
  spline S57 degree 3 poles (31.2925, -55.4696) (31.2371, -55.5125) (31.1199, -55.603) (30.9716, -55.612) (30.8935, -55.6166) knots 0 0 0 0 0.020535 0.043408 0.043408 0.043408 0.043408
  line L470 (30.8935, -55.6166) -> (30.3055, -55.6166)
  spline S58 degree 3 poles (30.3055, -55.6166) (30.1521, -55.6021) (29.8436, -55.5727) (29.6059, -55.3737) (29.4865, -55.2736) knots 0 0 0 0 0.045098 0.090676 0.090676 0.090676 0.090676
  spline S59 degree 3 poles (29.4865, -55.2736) (29.3865, -55.1542) (29.1874, -54.9166) (29.1581, -54.6081) (29.1435, -54.4546) knots 0 0 0 0 0.045579 0.090676 0.090676 0.090676 0.090676
  line L471 (29.1435, -54.4546) -> (29.1435, -51.5356)
  line L472 (29.1435, -51.5356) -> (30.3055, -51.5356)
  line L473 (30.3055, -51.5356) -> (30.3055, -54.4546)
  spline S60 degree 3 poles (30.3055, -54.4546) (30.3129, -54.5312) (30.3279, -54.6852) (30.4294, -54.8019) (30.4805, -54.8606) knots 0 0 0 0 0.02248 0.045204 0.045204 0.045204 0.045204
  spline S61 degree 3 poles (30.4805, -54.8606) (30.5398, -54.9117) (30.6588, -55.0141) (30.8151, -55.0284) (30.8935, -55.0356) knots 0 0 0 0 0.022867 0.045862 0.045862 0.045862 0.045862
  spline S62 degree 3 poles (30.8935, -55.0356) (30.9705, -55.028) (31.1263, -55.0127) (31.246, -54.9117) (31.3065, -54.8606) knots 0 0 0 0 0.022651 0.045806 0.045806 0.045806 0.045806
  spline S63 degree 3 poles (31.3065, -54.8606) (31.3555, -54.8017) (31.4535, -54.6838) (31.4675, -54.5311) (31.4745, -54.4546) knots 0 0 0 0 0.022425 0.044871 0.044871 0.044871 0.044871
  line L474 (31.4745, -54.4546) -> (31.4745, -51.5356)
  line L475 (31.4745, -51.5356) -> (32.6435, -51.5356)
  line L476 (24.4745, -53.2856) -> (26.8055, -53.2856)
  line L477 (26.8055, -53.2856) -> (26.8055, -52.7046)
  spline S64 degree 3 poles (26.8055, -52.7046) (26.7983, -52.6278) (26.784, -52.4732) (26.6865, -52.3524) (26.6375, -52.2916) knots 0 0 0 0 0.022618 0.045479 0.045479 0.045479 0.045479
  spline S65 degree 3 poles (26.6375, -52.2916) (26.577, -52.2406) (26.4573, -52.1396) (26.3015, -52.1243) (26.2245, -52.1166) knots 0 0 0 0 0.023154 0.045806 0.045806 0.045806 0.045806
  line L478 (26.2245, -52.1166) -> (25.6365, -52.1166)
  spline S66 degree 3 poles (25.6365, -52.1166) (25.467, -52.1416) (25.1265, -52.1918) (25.0792, -52.5331) (25.0555, -52.7046) knots 0 0 0 0 0.045988 0.092418 0.092418 0.092418 0.092418
  line L479 (25.0555, -52.7046) -> (24.4745, -52.7046)
  spline S67 degree 3 poles (24.4745, -52.7046) (24.5469, -52.3639) (24.6847, -51.715) (25.33, -51.5934) (25.6365, -51.5356) knots 0 0 0 0 0.094665 0.180306 0.180306 0.180306 0.180306
  line L480 (25.6365, -51.5356) -> (26.8055, -51.5356)
  spline S68 degree 3 poles (26.8055, -51.5356) (26.9594, -51.5504) (27.2697, -51.5801) (27.5102, -51.7786) (27.6315, -51.8786) knots 0 0 0 0 0.04527 0.091283 0.091283 0.091283 0.091283
  spline S69 degree 3 poles (27.6315, -51.8786) (27.7315, -51.9987) (27.9314, -52.2386) (27.9601, -52.5494) (27.9745, -52.7046) knots 0 0 0 0 0.045723 0.091336 0.091336 0.091336 0.091336
  line L481 (27.9745, -52.7046) -> (27.9745, -54.4546)
  spline S70 degree 3 poles (27.9745, -54.4546) (27.9599, -54.6081) (27.9306, -54.9166) (27.7315, -55.1542) (27.6315, -55.2736) knots 0 0 0 0 0.045098 0.090676 0.090676 0.090676 0.090676
  spline S71 degree 3 poles (27.6315, -55.2736) (27.5102, -55.3737) (27.2697, -55.5722) (26.9594, -55.6019) (26.8055, -55.6166) knots 0 0 0 0 0.046013 0.091283 0.091283 0.091283 0.091283
  line L482 (26.8055, -55.6166) -> (25.6365, -55.6166)
  spline S72 degree 3 poles (25.6365, -55.6166) (25.4831, -55.6021) (25.1746, -55.5727) (24.9369, -55.3737) (24.8175, -55.2736) knots 0 0 0 0 0.045098 0.090676 0.090676 0.090676 0.090676
  spline S73 degree 3 poles (24.8175, -55.2736) (24.7174, -55.1542) (24.5184, -54.9166) (24.4891, -54.6081) (24.4745, -54.4546) knots 0 0 0 0 0.045579 0.090676 0.090676 0.090676 0.090676
  line L483 (24.4745, -54.4546) -> (24.4745, -53.2856)
  line L484 (26.8055, -53.8666) -> (25.6365, -53.8666)
  line L485 (25.6365, -53.8666) -> (25.6365, -54.4546)
  spline S74 degree 3 poles (25.6365, -54.4546) (25.6439, -54.5312) (25.6589, -54.6852) (25.7604, -54.8019) (25.8115, -54.8606) knots 0 0 0 0 0.02248 0.045204 0.045204 0.045204 0.045204
  spline S75 degree 3 poles (25.8115, -54.8606) (25.8708, -54.9117) (25.9898, -55.0141) (26.1461, -55.0284) (26.2245, -55.0356) knots 0 0 0 0 0.022867 0.045862 0.045862 0.045862 0.045862
  spline S76 degree 3 poles (26.2245, -55.0356) (26.3015, -55.028) (26.4573, -55.0127) (26.577, -54.9117) (26.6375, -54.8606) knots 0 0 0 0 0.022651 0.045806 0.045806 0.045806 0.045806
  spline S77 degree 3 poles (26.6375, -54.8606) (26.6865, -54.8017) (26.7845, -54.6838) (26.7985, -54.5311) (26.8055, -54.4546) knots 0 0 0 0 0.022425 0.044871 0.044871 0.044871 0.044871
  line L486 (26.8055, -54.4546) -> (26.8055, -53.8666)
  line L487 (20.9675, -53.8666) -> (20.9675, -54.4546)
  spline S78 degree 3 poles (20.9675, -54.4546) (20.9749, -54.5312) (20.9899, -54.6852) (21.0914, -54.8019) (21.1425, -54.8606) knots 0 0 0 0 0.02248 0.045204 0.045204 0.045204 0.045204
  spline S79 degree 3 poles (21.1425, -54.8606) (21.2018, -54.9117) (21.3208, -55.0141) (21.4771, -55.0284) (21.5555, -55.0356) knots 0 0 0 0 0.022867 0.045862 0.045862 0.045862 0.045862
  line L488 (21.5555, -55.0356) -> (22.1365, -55.0356)
  spline S80 degree 3 poles (22.1365, -55.0356) (22.2906, -55.0073) (22.6133, -54.9481) (22.6817, -54.624) (22.7175, -54.4546) knots 0 0 0 0 0.042956 0.089979 0.089979 0.089979 0.089979
  line L489 (22.7175, -54.4546) -> (23.3055, -54.4546)
  spline S81 degree 3 poles (23.3055, -54.4546) (23.2307, -54.7933) (23.0878, -55.4397) (22.4433, -55.5596) (22.1365, -55.6166) knots 0 0 0 0 0.094379 0.180125 0.180125 0.180125 0.180125
  line L490 (22.1365, -55.6166) -> (20.9675, -55.6166)
  spline S82 degree 3 poles (20.9675, -55.6166) (20.8141, -55.6021) (20.5056, -55.5727) (20.2679, -55.3737) (20.1485, -55.2736) knots 0 0 0 0 0.045098 0.090676 0.090676 0.090676 0.090676
  spline S83 degree 3 poles (20.1485, -55.2736) (20.0484, -55.1542) (19.8494, -54.9166) (19.8201, -54.6081) (19.8055, -54.4546) knots 0 0 0 0 0.045579 0.090676 0.090676 0.090676 0.090676
  line L491 (19.8055, -54.4546) -> (19.8055, -51.5356)
  line L492 (19.8055, -51.5356) -> (20.9675, -51.5356)
  line L493 (20.9675, -51.5356) -> (20.9675, -52.1166)
  spline S84 degree 3 poles (20.9675, -52.1166) (21.0053, -51.9473) (21.0776, -51.6233) (21.4011, -51.564) (21.5555, -51.5356) knots 0 0 0 0 0.047223 0.090343 0.090343 0.090343 0.090343
  line L494 (21.5555, -51.5356) -> (22.1365, -51.5356)
  spline S85 degree 3 poles (22.1365, -51.5356) (22.2904, -51.5504) (22.6007, -51.5801) (22.8412, -51.7786) (22.9625, -51.8786) knots 0 0 0 0 0.04527 0.091283 0.091283 0.091283 0.091283
  spline S86 degree 3 poles (22.9625, -51.8786) (23.0625, -51.9987) (23.2624, -52.2386) (23.2911, -52.5494) (23.3055, -52.7046) knots 0 0 0 0 0.045723 0.091336 0.091336 0.091336 0.091336
  spline S87 degree 3 poles (23.3055, -52.7046) (23.2909, -52.8581) (23.2616, -53.1666) (23.0625, -53.4042) (22.9625, -53.5236) knots 0 0 0 0 0.045098 0.090676 0.090676 0.090676 0.090676
  spline S88 degree 3 poles (22.9625, -53.5236) (22.8412, -53.6237) (22.6007, -53.8222) (22.2904, -53.8519) (22.1365, -53.8666) knots 0 0 0 0 0.046013 0.091283 0.091283 0.091283 0.091283
  line L495 (22.1365, -53.8666) -> (20.9675, -53.8666)
  line L496 (20.9675, -53.2856) -> (21.5555, -53.2856)
  spline S89 degree 3 poles (21.5555, -53.2856) (21.6325, -53.278) (21.7883, -53.2627) (21.908, -53.1617) (21.9685, -53.1106) knots 0 0 0 0 0.022651 0.045806 0.045806 0.045806 0.045806
  spline S90 degree 3 poles (21.9685, -53.1106) (22.0175, -53.0517) (22.1155, -52.9338) (22.1295, -52.7811) (22.1365, -52.7046) knots 0 0 0 0 0.022425 0.044871 0.044871 0.044871 0.044871
  spline S91 degree 3 poles (22.1365, -52.7046) (22.1293, -52.6278) (22.115, -52.4732) (22.0175, -52.3524) (21.9685, -52.2916) knots 0 0 0 0 0.022618 0.045479 0.045479 0.045479 0.045479
  spline S92 degree 3 poles (21.9685, -52.2916) (21.908, -52.2406) (21.7883, -52.1396) (21.6325, -52.1243) (21.5555, -52.1166) knots 0 0 0 0 0.023154 0.045806 0.045806 0.045806 0.045806
  spline S93 degree 3 poles (21.5555, -52.1166) (21.4771, -52.1239) (21.3208, -52.1382) (21.2018, -52.2406) (21.1425, -52.2916) knots 0 0 0 0 0.022995 0.045862 0.045862 0.045862 0.045862
  spline S94 degree 3 poles (21.1425, -52.2916) (21.0915, -52.3522) (20.9905, -52.4719) (20.9751, -52.6276) (20.9675, -52.7046) knots 0 0 0 0 0.023154 0.045806 0.045806 0.045806 0.045806
  line L497 (20.9675, -52.7046) -> (20.9675, -53.2856)
  line L498 (18.0485, -56.7856) -> (16.8865, -56.7856)
  line L499 (16.8865, -56.7856) -> (16.8865, -55.6166)
  line L500 (16.8865, -55.6166) -> (16.2985, -55.6166)
  line L501 (16.2985, -55.6166) -> (16.2985, -55.0356)
  line L502 (16.2985, -55.0356) -> (16.8865, -55.0356)
  line L503 (16.8865, -55.0356) -> (16.8865, -52.7046)
  spline S95 degree 3 poles (16.8865, -52.7046) (16.8802, -52.6159) (16.8682, -52.4463) (16.7526, -52.3226) (16.6975, -52.2636) knots 0 0 0 0 0.025811 0.049296 0.049296 0.049296 0.049296
  spline S96 degree 3 poles (16.6975, -52.2636) (16.6398, -52.221) (16.5366, -52.1446) (16.4102, -52.1252) (16.3545, -52.1166) knots 0 0 0 0 0.021129 0.037814 0.037814 0.037814 0.037814
  line L504 (16.3545, -52.1166) -> (16.2985, -52.1166)
  line L505 (16.2985, -52.1166) -> (16.2985, -51.5356)
  line L506 (16.2985, -51.5356) -> (16.8865, -51.5356)
  spline S97 degree 3 poles (16.8865, -51.5356) (17.0399, -51.5502) (17.3484, -51.5796) (17.586, -51.7786) (17.7055, -51.8786) knots 0 0 0 0 0.045098 0.090676 0.090676 0.090676 0.090676
  spline S98 degree 3 poles (17.7055, -51.8786) (17.8055, -51.9987) (18.0054, -52.2386) (18.0341, -52.5494) (18.0485, -52.7046) knots 0 0 0 0 0.045723 0.091337 0.091337 0.091337 0.091337
  line L507 (18.0485, -52.7046) -> (18.0485, -55.0356)
  line L508 (18.0485, -55.0356) -> (18.6365, -55.0356)
  line L509 (18.6365, -55.0356) -> (18.6365, -55.6166)
  line L510 (18.6365, -55.6166) -> (18.0485, -55.6166)
  line L511 (18.0485, -55.6166) -> (18.0485, -56.7856)
  line L512 (13.3865, -51.5356) -> (13.3865, -56.7856)
  line L513 (13.3865, -56.7856) -> (12.2175, -56.7856)
  line L514 (12.2175, -56.7856) -> (12.2175, -55.0356)
  spline S99 degree 3 poles (12.2175, -55.0356) (12.2041, -55.1242) (12.1798, -55.2849) (12.0802, -55.4124) (12.0355, -55.4696) knots 0 0 0 0 0.026315 0.047768 0.047768 0.047768 0.047768
  spline S100 degree 3 poles (12.0355, -55.4696) (11.9801, -55.5125) (11.8629, -55.603) (11.7146, -55.612) (11.6365, -55.6166) knots 0 0 0 0 0.020535 0.043407 0.043407 0.043407 0.043407
  line L515 (11.6365, -55.6166) -> (11.0485, -55.6166)
  spline S101 degree 3 poles (11.0485, -55.6166) (10.8951, -55.6021) (10.5866, -55.5727) (10.3489, -55.3737) (10.2295, -55.2736) knots 0 0 0 0 0.045098 0.090677 0.090677 0.090677 0.090677
  spline S102 degree 3 poles (10.2295, -55.2736) (10.1294, -55.1542) (9.9304, -54.9166) (9.9011, -54.6081) (9.8865, -54.4546) knots 0 0 0 0 0.045579 0.090676 0.090676 0.090676 0.090676
  line L516 (9.8865, -54.4546) -> (9.8865, -52.7046)
  spline S103 degree 3 poles (9.8865, -52.7046) (9.9012, -52.5508) (9.931, -52.2405) (10.1295, -51.9999) (10.2295, -51.8786) knots 0 0 0 0 0.04527 0.091283 0.091283 0.091283 0.091283
  spline S104 degree 3 poles (10.2295, -51.8786) (10.3489, -51.7786) (10.5866, -51.5796) (10.8951, -51.5502) (11.0485, -51.5356) knots 0 0 0 0 0.045579 0.090677 0.090677 0.090677 0.090677
  line L517 (11.0485, -51.5356) -> (13.3865, -51.5356)
  line L518 (12.2175, -52.1166) -> (11.6365, -52.1166)
  spline S105 degree 3 poles (11.6365, -52.1166) (11.5581, -52.1239) (11.4018, -52.1382) (11.2828, -52.2406) (11.2235, -52.2916) knots 0 0 0 0 0.022995 0.045862 0.045862 0.045862 0.045862
  spline S106 degree 3 poles (11.2235, -52.2916) (11.1725, -52.3522) (11.0715, -52.4719) (11.0561, -52.6276) (11.0485, -52.7046) knots 0 0 0 0 0.023154 0.045806 0.045806 0.045806 0.045806
  line L519 (11.0485, -52.7046) -> (11.0485, -54.4546)